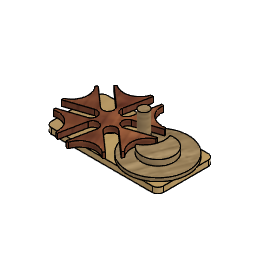
Mechanism v1 (Autodesk Fusion 360 design; units mm, degrees)
Autodesk Fusion 360 part; units mm, degrees
sketch "Sketch1" plane through (0, 0, 0) normal (0, 0, 1) x (1, 0, 0)
  line L0 (-45, 25) -> (45, 25)
  line L1 (50, 20) -> (50, -20)
  line L2 (45, -25) -> (-45, -25)
  line L3 (-50, -20) -> (-50, 20)
  arc A0 (-45, 25) -> (-50, 20) centre (-45, 20) ccw
  arc A1 (50, 20) -> (45, 25) centre (45, 20) ccw
  arc A2 (45, -25) -> (50, -20) centre (45, -20) ccw
  arc A3 (-50, -20) -> (-45, -25) centre (-45, -20) ccw
  dimension "d1" = 5
  constraint horizontal L0
  constraint vertical L1
  constraint horizontal L2
  constraint vertical L3
  constraint tangent L0 A0
  constraint tangent L3 A0
  constraint tangent L0 A1
  constraint tangent L1 A1
  constraint equal A0 A1
  constraint tangent L1 A2
  constraint tangent L2 A2
  constraint equal A0 A2
  constraint tangent L2 A3
  constraint tangent L3 A3
  constraint equal A0 A3
  measures "d1" radius of A0
extrude "Extrude1" add sketch "Sketch1" along normal blind 5 makes body 1
sketch "Sketch2" plane through (0, 0, 5) normal (0, 0, 1) x (-1, 0, 0)
  arc A0 (45, -25) -> (50, -20) centre (45, -20) ccw
  line L0 (50, -20) -> (50, 20)
  arc A1 (50, 20) -> (45, 25) centre (45, 20) ccw
  line L1 (45, 25) -> (-45, 25)
  arc A2 (-45, 25) -> (-50, 20) centre (-45, 20) ccw
  line L2 (-50, 20) -> (-50, -20)
  arc A3 (-50, -20) -> (-45, -25) centre (-45, -20) ccw
  line L3 (-45, -25) -> (45, -25)
  circle A4 centre (-25, 0) radius 27.2029
extrude "Extrude1'" add sketch "Sketch2" along normal blind 3 separate body contours L3 A4 | L1 L2 L3 A4 | L2 A4 | L1 A4 makes body 2 in component "Crank"
sketch "Sketch3" plane through (0, 0, 8) normal (0, 0, 1) x (-1, 0, 0)
  circle A0 centre (-25, 0) radius 27.2029
  circle A1 centre (-25, 0) radius 14.3178
  circle A2 centre (-47, 0) radius 15.6525
  constraint concentric A0 A1
extrude "Extrude2" add sketch "Sketch3" along normal blind 5 contours A1 A2 picked at (-24.968, 2.7723) bodies 2 in component "Crank"
sketch "Sketch4" plane through (0, 0, 8) normal (0, 0, 1) x (-1, 0, 0)
  arc A0 (-35.0909, -10.1574) -> (-35.0909, 10.1574) centre (-47, 0) ccw
  arc A1 (-35.0909, -10.1574) -> (-35.0909, 10.1574) centre (-25, 0) ccw
  circle A2 centre (-25, 0) radius 27.2029
  circle A3 centre (-47, 0) radius 4.5
  dimension "d8" = 9
  constraint concentric A0 A3
  measures "d8" diameter of A3
sketch "Sketch5" plane through (0, 0, 8) normal (0, 0, 1) x (-1, 0, 0)
extrude "Extrude3" add sketch "Sketch4" along normal blind 20 contours A3 bodies 2 in component "Crank"
sketch "Sketch1 (2)" plane through (0, 0, 5) normal (0, 0, -1) x (1, 0, 0) in component "Crank"
  circle A0 centre (25, 0) radius 27.2029
  circle A1 centre (25, 0) radius 3.6056
  constraint concentric A0 A1
extrude "Extrude4" add sketch "Sketch1 (2)" along normal blind 3 contours A1 bodies 2 in component "Crank"
sketch "Sketch2 (2)" plane through (0, 0, 5) normal (0, 0, 1) x (-1, 0, 0) in component "Crank"
  arc A0 (45, -25) -> (50, -20) centre (45, -20) ccw
  line L0 (50, -20) -> (50, 20)
  arc A1 (50, 20) -> (45, 25) centre (45, 20) ccw
  line L1 (45, 25) -> (-45, 25)
  arc A2 (-45, 25) -> (-50, 20) centre (-45, 20) ccw
  line L2 (-50, 20) -> (-50, -20)
  arc A3 (-50, -20) -> (-45, -25) centre (-45, -20) ccw
  line L3 (-45, -25) -> (45, -25)
  circle A4 centre (-25, 0) radius 5
extrude "Extrude2'" cut sketch "Sketch2 (2)" against normal blind 3 contours A4 bodies 1
extrude "Extrude5" cut sketch "Sketch2 (2)" against normal blind 3 contours A4 bodies 2 in component "Crank"
sketch "Sketch6" plane through (0, 0, 8) normal (0, 0, 1) x (-1, 0, 0)
  circle A0 centre (-47, 0) radius 4.5
  arc A1 (-35.0909, -10.1574) -> (-35.0909, 10.1574) centre (-47, 0) ccw
  arc A2 (-35.0909, -10.1574) -> (-35.0909, 10.1574) centre (-25, 0) ccw
  circle A3 centre (-25, 0) radius 27.2029
  circle A4 centre (15, 0) radius 36.685
  circle A5 centre (-6.0882, -30.018) radius 36.685
  circle A6 centre (30.4523, -33.2719) radius 36.685
  circle A7 centre (51.5405, -3.2539) radius 36.685
  circle A8 centre (36.0882, 30.018) radius 36.685
  circle A9 centre (-0.4523, 33.2719) radius 36.685
  circle A10 centre (-21.5405, 3.2539) radius 36.685
  line L0 (-6.0882, -30.018) -> (15, 0)
  line L1 (30.4523, -33.2719) -> (15, 0)
  line L2 (51.5405, -3.2539) -> (15, 0)
  line L3 (36.0882, 30.018) -> (15, 0)
  line L4 (-0.4523, 33.2719) -> (15, 0)
  line L5 (-21.5405, 3.2539) -> (15, 0)
  line L6 (-21.9839, -1.7264) -> (1.7355, -3.8386)
  arc A11 (1.7355, -3.8386) -> (2.6225, 6.122) centre (2.179, 1.1417) ccw
  line L7 (2.6225, 6.122) -> (-21.097, 8.2342)
  arc A12 (-21.097, 8.2342) -> (-21.9839, -1.7264) centre (-21.5405, 3.2539) ccw
  line L8 (-21.5405, 3.2539) -> (2.179, 1.1417) construction
  line L9 (-1.9969, -32.8922) -> (11.6379, -13.4839)
  arc A13 (11.6379, -13.4839) -> (3.4552, -7.7354) centre (7.5465, -10.6096) ccw
  line L10 (3.4552, -7.7354) -> (-10.1795, -27.1438)
  arc A14 (-10.1795, -27.1438) -> (-1.9969, -32.8922) centre (-6.0882, -30.018) ccw
  line L11 (-6.0882, -30.018) -> (7.5465, -10.6096) construction
  line L12 (34.9871, -31.1658) -> (24.9963, -9.6536)
  arc A15 (24.9963, -9.6536) -> (15.9267, -13.8658) centre (20.4615, -11.7597) ccw
  line L13 (15.9267, -13.8658) -> (25.9175, -35.378)
  arc A16 (25.9175, -35.378) -> (34.9871, -31.1658) centre (30.4523, -33.2719) ccw
  line L14 (30.4523, -33.2719) -> (20.4615, -11.7597) construction
  line L15 (51.9839, 1.7264) -> (28.3584, 3.8302)
  arc A17 (28.3584, 3.8302) -> (27.4715, -6.1304) centre (27.9149, -1.1501) ccw
  line L16 (27.4715, -6.1304) -> (51.097, -8.2342)
  arc A18 (51.097, -8.2342) -> (51.9839, 1.7264) centre (51.5405, -3.2539) ccw
  line L17 (51.5405, -3.2539) -> (27.9149, -1.1501) construction
  line L18 (31.9969, 32.8922) -> (18.3621, 13.4839)
  arc A19 (18.3621, 13.4839) -> (26.5448, 7.7354) centre (22.4535, 10.6096) ccw
  line L19 (26.5448, 7.7354) -> (40.1795, 27.1438)
  arc A20 (40.1795, 27.1438) -> (31.9969, 32.8922) centre (36.0882, 30.018) ccw
  line L20 (36.0882, 30.018) -> (22.4535, 10.6096) construction
  line L21 (-4.9871, 31.1658) -> (5.0037, 9.6536)
  arc A21 (5.0037, 9.6536) -> (14.0733, 13.8658) centre (9.5385, 11.7597) ccw
  line L22 (14.0733, 13.8658) -> (4.0825, 35.378)
  arc A22 (4.0825, 35.378) -> (-4.9871, 31.1658) centre (-0.4523, 33.2719) ccw
  line L23 (-0.4523, 33.2719) -> (9.5385, 11.7597) construction
  dimension "d17" = 10
  dimension "d18" = 23.719
  dimension "d19" = 10
  dimension "d20" = 10
  dimension "d21" = 10
  dimension "d22" = 10
  dimension "d23" = 23.719
  dimension "d24" = 10
  constraint coincident A4 A5.centre
  constraint coincident A4.centre A5
  constraint coincident A4 A6.centre
  constraint coincident A5 A6.centre
  constraint coincident A4.centre A6
  constraint coincident A4 A7.centre
  constraint coincident A6 A7.centre
  constraint coincident A4.centre A7
  constraint coincident A4 A8.centre
  constraint coincident A7 A8.centre
  constraint coincident A4.centre A8
  constraint coincident A8 A9.centre
  constraint coincident A4 A9.centre
  constraint coincident A4.centre A9
  constraint coincident A4 A10.centre
  constraint coincident A5 A10.centre
  constraint coincident A4.centre A10
  constraint coincident A5.centre L0.start
  constraint coincident A4.centre L0.end
  constraint coincident A6.centre L1.start
  constraint coincident A7.centre L2.start
  constraint coincident A8.centre L3.start
  constraint coincident A9.centre L4.start
  constraint coincident A10.centre L5.start
  constraint tangent L6 A11
  constraint tangent A11 L7
  constraint parallel L6 L7
  constraint tangent L7 A12
  constraint tangent L6 A12
  constraint coincident L5 A11.centre
  constraint coincident A3 A11.centre
  constraint parallel L5 L8
  constraint tangent L9 A13
  constraint tangent A13 L10
  constraint parallel L9 L10
  constraint tangent L10 A14
  constraint tangent L9 A14
  constraint coincident L0 A13.centre
  constraint parallel L0 L11
  constraint tangent L12 A15
  constraint tangent A15 L13
  constraint parallel L12 L13
  constraint tangent L13 A16
  constraint tangent L12 A16
  constraint parallel L1 L14
  constraint tangent L15 A17
  constraint tangent A17 L16
  constraint parallel L15 L16
  constraint tangent L16 A18
  constraint tangent L15 A18
  constraint parallel L2 L17
  constraint tangent L18 A19
  constraint tangent A19 L19
  constraint parallel L18 L19
  constraint tangent L19 A20
  constraint tangent L18 A20
  constraint parallel L3 L20
  constraint tangent L21 A21
  constraint tangent A21 L22
  constraint parallel L21 L22
  constraint tangent L22 A22
  constraint tangent L21 A22
  constraint coincident L4 A21.centre
  constraint parallel L4 L23
  measures "d17" diameter of A11
  measures "d18" distance of A5.centre A13.centre
  measures "d19" diameter of A13
  measures "d20" diameter of A15
  measures "d21" diameter of A17
  measures "d22" diameter of A19
  measures "d23" distance of A9.centre A21.centre
  measures "d24" diameter of A21
extrude "Extrude1''" add sketch "Sketch6" along normal blind 5 separate body contours A2 A4 L6 | A2 A3 A4 L6 A11 | A3 A4 A6 A9 A11 A13 L10 | A2 A3 A4 L7 | A2 A4 L7 | A3 A4 A5 A8 A11 L7 L21 A21 | A9 L5 A11 | A4 A5 A8 L12 A15 A17 L16 | A5 L5 A11 | A4 A6 A9 L15 A17 A19 L19 | A6 L0 A13 | A4 A7 A10 L18 A19 A21 L22 | A7 L1 A15 | A8 L2 A17 | A9 L3 A19 | A10 L4 A21 | A4 A7 A10 L9 A13 A15 L13 | A10 L0 A13 | A5 L1 A15 | A6 L2 A17 | A7 L3 A19 | A8 L4 A21 picked at (10.2053, -3.8088) picked at (15.9012, -6.0568) picked at (20.6959, -2.2479) picked at (19.7947, 3.8088) picked at (13.9503, 5.3986) picked at (13.0428, -5.8022) picked at (19.0463, -4.5961) picked at (21.0035, 1.2061) picked at (16.9572, 5.8022) picked at (10.9537, 4.5961) makes body 3 in component "Star gear"
move_body "Move1" bodies 3 to x (1, 0, 0) y (0, 1, 0) z (0, 0, 1) at (-3, 0, 0) in component "Star gear"
move_body "Move2" bodies 3 to x (0.906308, -0.422618, 0) y (0.422618, 0.906308, 0) z (0, 0, 1) at (-1.6865, -7.6071, 0) in component "Star gear"
sketch "Sketch7" plane through (0, 0, 13) normal (0, 0, 1) x (-1, 0, 0)
  arc A0 (13.0563, 36.3504) -> (-10.9388, 22.5463) centre (18, 0) ccw
  line L0 (-10.9388, 22.5463) -> (9.3694, 10.7794)
  arc A1 (4.356, 2.1269) -> (9.3694, 10.7794) centre (6.8627, 6.4531) ccw
  line L1 (4.356, 2.1269) -> (-15.9522, 13.8938)
  arc A2 (-15.9522, 13.8938) -> (-15.9951, -13.7886) centre (18, 0) ccw
  line L2 (-15.9951, -13.7886) -> (4.2678, -2.1316)
  arc A3 (9.2543, -10.7996) -> (4.2678, -2.1316) centre (6.7611, -6.4656) ccw
  line L3 (9.2543, -10.7996) -> (-11.0085, -22.4566)
  arc A4 (-11.0085, -22.4566) -> (12.9437, -36.3349) centre (18, 0) ccw
  line L4 (12.9437, -36.3349) -> (12.9799, -12.9583)
  arc A5 (22.9799, -12.9738) -> (12.9799, -12.9583) centre (17.9799, -12.966) ccw
  line L5 (22.9799, -12.9738) -> (22.9437, -36.3504)
  arc A6 (22.9437, -36.3504) -> (46.9388, -22.5463) centre (18, 0) ccw
  line L6 (46.9388, -22.5463) -> (26.7122, -10.8267)
  arc A7 (31.7256, -2.1741) -> (26.7122, -10.8267) centre (29.2189, -6.5004) ccw
  line L7 (31.7256, -2.1741) -> (51.9522, -13.8938)
  arc A8 (51.9522, -13.8938) -> (51.9951, 13.7886) centre (18, 0) ccw
  line L8 (51.9951, 13.7886) -> (31.7322, 2.1316)
  arc A9 (26.7457, 10.7996) -> (31.7322, 2.1316) centre (29.2389, 6.4656) ccw
  line L9 (26.7457, 10.7996) -> (47.0085, 22.4566)
  arc A10 (47.0085, 22.4566) -> (23.0563, 36.3349) centre (18, 0) ccw
  line L10 (23.0563, 36.3349) -> (23.0201, 12.9583)
  arc A11 (13.0201, 12.9738) -> (23.0201, 12.9583) centre (18.0201, 12.966) ccw
  line L11 (13.0201, 12.9738) -> (13.0563, 36.3504)
  circle A12 centre (-10.587, 0.0568) radius 14.6
  circle A13 centre (-25.1869, 0.0083) radius 14.6433
  circle A14 centre (18, 0) radius 36.685
  dimension "d27" = 29.2
  constraint coincident A12 A13.centre
  constraint concentric A0 A14
  measures "d27" diameter of A12
extrude "Extrude2''" cut sketch "Sketch7" against normal blind 5 contours A2 A13 A14 bodies 3 in component "Star gear"
move_body "Move3" bodies 3 to x (0.5, 0.866025, 0) y (-0.866025, 0.5, 0) z (0, 0, 1) at (-9, 15.5885, 0) in component "Star gear"
sketch "Sketch8" plane through (0, 0, 13) normal (0, 0, 1) x (-1, 0, 0)
  arc A0 (10.9765, -36.0064) -> (-9.68, -24.0751) centre (-3.6007, -37.3968) ccw
  arc A1 (10.9765, -36.0064) -> (12.9437, -36.3349) centre (18, 0) ccw
  line L0 (12.9437, -36.3349) -> (12.9799, -12.9583)
  arc A2 (22.9799, -12.9738) -> (12.9799, -12.9583) centre (17.9799, -12.966) ccw
  line L1 (22.9799, -12.9738) -> (22.9437, -36.3504)
  arc A3 (22.9437, -36.3504) -> (46.9388, -22.5463) centre (18, 0) ccw
  line L2 (46.9388, -22.5463) -> (26.7122, -10.8267)
  arc A4 (31.7256, -2.1741) -> (26.7122, -10.8267) centre (29.2189, -6.5004) ccw
  line L3 (31.7256, -2.1741) -> (51.9522, -13.8938)
  arc A5 (51.9522, -13.8938) -> (51.9951, 13.7886) centre (18, 0) ccw
  line L4 (51.9951, 13.7886) -> (31.7322, 2.1316)
  arc A6 (26.7457, 10.7996) -> (31.7322, 2.1316) centre (29.2389, 6.4656) ccw
  line L5 (26.7457, 10.7996) -> (47.0085, 22.4566)
  arc A7 (47.0085, 22.4566) -> (23.0563, 36.3349) centre (18, 0) ccw
  line L6 (23.0563, 36.3349) -> (23.0201, 12.9583)
  arc A8 (13.0201, 12.9738) -> (23.0201, 12.9583) centre (18.0201, 12.966) ccw
  line L7 (13.0201, 12.9738) -> (13.0563, 36.3504)
  arc A9 (13.0563, 36.3504) -> (-10.9388, 22.5463) centre (18, 0) ccw
  line L8 (-10.9388, 22.5463) -> (9.2878, 10.8267)
  arc A10 (4.2744, 2.1741) -> (9.2878, 10.8267) centre (6.7811, 6.5004) ccw
  line L9 (4.2744, 2.1741) -> (-15.9522, 13.8938)
  arc A11 (-15.9522, 13.8938) -> (-15.9951, -13.7886) centre (18, 0) ccw
  line L10 (-15.9951, -13.7886) -> (4.3495, -2.0846)
  arc A12 (9.3361, -10.7526) -> (4.3495, -2.0846) centre (6.8428, -6.4186) ccw
  line L11 (9.3361, -10.7526) -> (-11.0085, -22.4566)
  arc A13 (-11.0085, -22.4566) -> (-9.68, -24.0751) centre (18, 0) ccw
  circle A14 centre (-10.7, 0) radius 14.6
  circle A15 centre (-25.2997, -0.0928) radius 14.75
  dimension "d30" = 29.2
  dimension "d31" = 29.5
  constraint coincident A14 A15.centre
  measures "d30" diameter of A14
  measures "d31" diameter of A15
extrude "Extrude3'" cut sketch "Sketch8" against normal blind 5 contours A11 A15 bodies 3 in component "Star gear"
move_body "Move4" bodies 3 to x (0.5, 0.866025, 0) y (-0.866025, 0.5, 0) z (0, 0, 1) at (-9, 15.5885, 0) in component "Star gear"
sketch "Sketch9" plane through (0, 0, 13) normal (0, 0, 1) x (-1, 0, 0)
  arc A0 (11.1026, -36.0308) -> (-9.6518, -24.1075) centre (-3.5695, -37.545) ccw
  arc A1 (11.1026, -36.0308) -> (12.9437, -36.3349) centre (18, 0) ccw
  line L0 (12.9437, -36.3349) -> (12.9801, -12.864)
  arc A2 (22.9801, -12.8795) -> (12.9801, -12.864) centre (17.9801, -12.8717) ccw
  line L1 (22.9801, -12.8795) -> (22.9437, -36.3504)
  arc A3 (22.9437, -36.3504) -> (25.0097, -36.0091) centre (18, 0) ccw
  arc A4 (45.6707, -24.0858) -> (25.0097, -36.0091) centre (39.5862, -37.4051) ccw
  arc A5 (45.6707, -24.0858) -> (46.9388, -22.5463) centre (18, 0) ccw
  line L2 (46.9388, -22.5463) -> (26.7122, -10.8267)
  arc A6 (31.7256, -2.1741) -> (26.7122, -10.8267) centre (29.2189, -6.5004) ccw
  line L3 (31.7256, -2.1741) -> (51.9522, -13.8938)
  arc A7 (51.9522, -13.8938) -> (51.9951, 13.7886) centre (18, 0) ccw
  line L4 (51.9951, 13.7886) -> (31.7322, 2.1316)
  arc A8 (26.7457, 10.7996) -> (31.7322, 2.1316) centre (29.2389, 6.4656) ccw
  line L5 (26.7457, 10.7996) -> (47.0085, 22.4566)
  arc A9 (47.0085, 22.4566) -> (23.0563, 36.3349) centre (18, 0) ccw
  line L6 (23.0563, 36.3349) -> (23.0201, 12.9583)
  arc A10 (13.0201, 12.9738) -> (23.0201, 12.9583) centre (18.0201, 12.966) ccw
  line L7 (13.0201, 12.9738) -> (13.0563, 36.3504)
  arc A11 (13.0563, 36.3504) -> (-10.9388, 22.5463) centre (18, 0) ccw
  line L8 (-10.9388, 22.5463) -> (9.2878, 10.8267)
  arc A12 (4.2744, 2.1741) -> (9.2878, 10.8267) centre (6.7811, 6.5004) ccw
  line L9 (4.2744, 2.1741) -> (-15.9522, 13.8938)
  arc A13 (-15.9522, 13.8938) -> (-15.9951, -13.7886) centre (18, 0) ccw
  line L10 (-15.9951, -13.7886) -> (4.2678, -2.1316)
  arc A14 (9.2543, -10.7996) -> (4.2678, -2.1316) centre (6.7611, -6.4656) ccw
  line L11 (9.2543, -10.7996) -> (-11.0085, -22.4566)
  arc A15 (-11.0085, -22.4566) -> (-9.6518, -24.1075) centre (18, 0) ccw
  circle A16 centre (-24.9492, 0.0568) radius 14.5
  dimension "d34" = 29
  measures "d34" diameter of A16
extrude "Extrude4'" cut sketch "Sketch9" against normal blind 5 contours A13 A16 picked at (-15.8862, 0.0512) bodies 3 in component "Star gear"
move_body "Move5" bodies 3 to x (0.5, 0.866025, 0) y (-0.866025, 0.5, 0) z (0, 0, 1) at (-9, 15.5885, 0) in component "Star gear"
sketch "Sketch10" plane through (0, 0, 13) normal (0, 0, 1) x (-1, 0, 0)
  arc A0 (10.929, -35.9971) -> (-9.7026, -24.0491) centre (-3.5238, -37.1667) ccw
  arc A1 (10.929, -35.9971) -> (12.9437, -36.3349) centre (18, 0) ccw
  line L0 (12.9437, -36.3349) -> (12.9799, -12.9583)
  arc A2 (22.9799, -12.9738) -> (12.9799, -12.9583) centre (17.9799, -12.966) ccw
  line L1 (22.9799, -12.9738) -> (22.9437, -36.3504)
  arc A3 (22.9437, -36.3504) -> (25.0518, -36.0009) centre (18, 0) ccw
  arc A4 (45.7549, -23.9887) -> (25.0518, -36.0009) centre (39.7302, -37.4522) ccw
  arc A5 (45.7549, -23.9887) -> (46.9388, -22.5463) centre (18, 0) ccw
  line L2 (46.9388, -22.5463) -> (26.6306, -10.7794)
  arc A6 (31.644, -2.1269) -> (26.6306, -10.7794) centre (29.1373, -6.4531) ccw
  line L3 (31.644, -2.1269) -> (51.9522, -13.8938)
  arc A7 (51.9522, -13.8938) -> (52.6896, -11.934) centre (18, 0) ccw
  arc A8 (52.6942, 11.9206) -> (52.6896, -11.934) centre (61.1869, -0.0083) ccw
  arc A9 (52.6942, 11.9206) -> (51.9951, 13.7886) centre (18, 0) ccw
  line L4 (51.9951, 13.7886) -> (31.7322, 2.1316)
  arc A10 (26.7457, 10.7996) -> (31.7322, 2.1316) centre (29.2389, 6.4656) ccw
  line L5 (26.7457, 10.7996) -> (47.0085, 22.4566)
  arc A11 (47.0085, 22.4566) -> (23.0563, 36.3349) centre (18, 0) ccw
  line L6 (23.0563, 36.3349) -> (23.0201, 12.9583)
  arc A12 (13.0201, 12.9738) -> (23.0201, 12.9583) centre (18.0201, 12.966) ccw
  line L7 (13.0201, 12.9738) -> (13.0563, 36.3504)
  arc A13 (13.0563, 36.3504) -> (-10.9388, 22.5463) centre (18, 0) ccw
  line L8 (-10.9388, 22.5463) -> (9.2878, 10.8267)
  arc A14 (4.2744, 2.1741) -> (9.2878, 10.8267) centre (6.7811, 6.5004) ccw
  line L9 (4.2744, 2.1741) -> (-15.9522, 13.8938)
  arc A15 (-15.9522, 13.8938) -> (-15.9951, -13.7886) centre (18, 0) ccw
  line L10 (-15.9951, -13.7886) -> (4.2678, -2.1316)
  arc A16 (9.2543, -10.7996) -> (4.2678, -2.1316) centre (6.7611, -6.4656) ccw
  line L11 (9.2543, -10.7996) -> (-11.0085, -22.4566)
  arc A17 (-11.0085, -22.4566) -> (-9.7026, -24.0491) centre (18, 0) ccw
  circle A18 centre (-25, 0) radius 14.5
  dimension "d37" = 29
  measures "d37" diameter of A18
extrude "Extrude5'" cut sketch "Sketch10" against normal blind 5 contours A15 A18 picked at (-15.9034, 0) bodies 3 in component "Star gear"
move_body "Move6" bodies 3 to x (0.5, 0.866025, 0) y (-0.866025, 0.5, 0) z (0, 0, 1) at (-9, 15.5885, 0) in component "Star gear"
sketch "Sketch11" plane through (0, 0, 13) normal (0, 0, 1) x (-1, 0, 0)
  arc A0 (10.947, -36.0007) -> (-9.651, -24.1084) centre (-3.5, -37.2391) ccw
  arc A1 (10.947, -36.0007) -> (12.9437, -36.3349) centre (18, 0) ccw
  line L0 (12.9437, -36.3349) -> (12.9799, -12.9583)
  arc A2 (22.9799, -12.9738) -> (12.9799, -12.9583) centre (17.9799, -12.966) ccw
  line L1 (22.9799, -12.9738) -> (22.9437, -36.3504)
  arc A3 (22.9437, -36.3504) -> (24.9758, -36.0157) centre (18, 0) ccw
  arc A4 (45.6389, -24.1222) -> (24.9758, -36.0157) centre (39.4254, -37.2235) ccw
  arc A5 (45.6389, -24.1222) -> (46.9388, -22.5463) centre (18, 0) ccw
  line L2 (46.9388, -22.5463) -> (26.7122, -10.8267)
  arc A6 (31.7256, -2.1741) -> (26.7122, -10.8267) centre (29.2189, -6.5004) ccw
  line L3 (31.7256, -2.1741) -> (51.9522, -13.8938)
  arc A7 (51.9522, -13.8938) -> (52.7036, -11.8934) centre (18, 0) ccw
  arc A8 (52.6523, 12.0421) -> (52.7036, -11.8934) centre (61.2997, 0.0928) ccw
  arc A9 (52.6523, 12.0421) -> (51.9951, 13.7886) centre (18, 0) ccw
  line L4 (51.9951, 13.7886) -> (31.6505, 2.0846)
  arc A10 (26.6639, 10.7526) -> (31.6505, 2.0846) centre (29.1572, 6.4186) ccw
  line L5 (26.6639, 10.7526) -> (47.0085, 22.4566)
  arc A11 (47.0085, 22.4566) -> (45.68, 24.0751) centre (18, 0) ccw
  arc A12 (25.0235, 36.0064) -> (45.68, 24.0751) centre (39.6007, 37.3968) ccw
  arc A13 (25.0235, 36.0064) -> (23.0563, 36.3349) centre (18, 0) ccw
  line L6 (23.0563, 36.3349) -> (23.0201, 12.9583)
  arc A14 (13.0201, 12.9738) -> (23.0201, 12.9583) centre (18.0201, 12.966) ccw
  line L7 (13.0201, 12.9738) -> (13.0563, 36.3504)
  arc A15 (13.0563, 36.3504) -> (-10.9388, 22.5463) centre (18, 0) ccw
  line L8 (-10.9388, 22.5463) -> (9.2878, 10.8267)
  arc A16 (4.2744, 2.1741) -> (9.2878, 10.8267) centre (6.7811, 6.5004) ccw
  line L9 (4.2744, 2.1741) -> (-15.9522, 13.8938)
  arc A17 (-15.9522, 13.8938) -> (-15.9951, -13.7886) centre (18, 0) ccw
  line L10 (-15.9951, -13.7886) -> (4.2678, -2.1316)
  arc A18 (9.2543, -10.7996) -> (4.2678, -2.1316) centre (6.7611, -6.4656) ccw
  line L11 (9.2543, -10.7996) -> (-11.0085, -22.4566)
  arc A19 (-11.0085, -22.4566) -> (-9.651, -24.1084) centre (18, 0) ccw
  circle A20 centre (-25, 0) radius 14.5
  dimension "d40" = 29
  measures "d40" diameter of A20
extrude "Extrude6" cut sketch "Sketch11" against normal blind 5 contours A17 A20 picked at (-15.9034, 0) bodies 3 in component "Star gear"
move_body "Move7" bodies 3 to x (0.5, 0.866025, 0) y (-0.866025, 0.5, 0) z (0, 0, 1) at (-9, 15.5885, 0) in component "Star gear"
sketch "Sketch12" plane through (0, 0, 13) normal (0, 0, 1) x (-1, 0, 0)
  arc A0 (10.947, -36.0007) -> (-9.651, -24.1084) centre (-3.5, -37.2391) ccw
  arc A1 (10.947, -36.0007) -> (12.9437, -36.3349) centre (18, 0) ccw
  line L0 (12.9437, -36.3349) -> (12.9799, -12.9583)
  arc A2 (22.9799, -12.9738) -> (12.9799, -12.9583) centre (17.9799, -12.966) ccw
  line L1 (22.9799, -12.9738) -> (22.9437, -36.3504)
  arc A3 (22.9437, -36.3504) -> (25.053, -36.0007) centre (18, 0) ccw
  arc A4 (45.651, -24.1084) -> (25.053, -36.0007) centre (39.5, -37.2391) ccw
  arc A5 (45.651, -24.1084) -> (46.9388, -22.5463) centre (18, 0) ccw
  line L2 (46.9388, -22.5463) -> (26.7122, -10.8267)
  arc A6 (31.7256, -2.1741) -> (26.7122, -10.8267) centre (29.2189, -6.5004) ccw
  line L3 (31.7256, -2.1741) -> (51.9522, -13.8938)
  arc A7 (51.9522, -13.8938) -> (52.6784, -11.9666) centre (18, 0) ccw
  arc A8 (52.7099, 11.8749) -> (52.6784, -11.9666) centre (60.9492, -0.0568) ccw
  arc A9 (52.7099, 11.8749) -> (51.9951, 13.7886) centre (18, 0) ccw
  line L4 (51.9951, 13.7886) -> (31.7322, 2.1316)
  arc A10 (26.7457, 10.7996) -> (31.7322, 2.1316) centre (29.2389, 6.4656) ccw
  line L5 (26.7457, 10.7996) -> (47.0085, 22.4566)
  arc A11 (47.0085, 22.4566) -> (45.6518, 24.1075) centre (18, 0) ccw
  arc A12 (24.8974, 36.0308) -> (45.6518, 24.1075) centre (39.5695, 37.545) ccw
  arc A13 (24.8974, 36.0308) -> (23.0563, 36.3349) centre (18, 0) ccw
  line L6 (23.0563, 36.3349) -> (23.0199, 12.864)
  arc A14 (13.0199, 12.8795) -> (23.0199, 12.864) centre (18.0199, 12.8717) ccw
  line L7 (13.0199, 12.8795) -> (13.0563, 36.3504)
  arc A15 (13.0563, 36.3504) -> (10.9903, 36.0091) centre (18, 0) ccw
  arc A16 (-9.6707, 24.0858) -> (10.9903, 36.0091) centre (-3.5862, 37.4051) ccw
  arc A17 (-9.6707, 24.0858) -> (-10.9388, 22.5463) centre (18, 0) ccw
  line L8 (-10.9388, 22.5463) -> (9.2878, 10.8267)
  arc A18 (4.2744, 2.1741) -> (9.2878, 10.8267) centre (6.7811, 6.5004) ccw
  line L9 (4.2744, 2.1741) -> (-15.9522, 13.8938)
  arc A19 (-15.9522, 13.8938) -> (-15.9951, -13.7886) centre (18, 0) ccw
  line L10 (-15.9951, -13.7886) -> (4.2678, -2.1316)
  arc A20 (9.2543, -10.7996) -> (4.2678, -2.1316) centre (6.7611, -6.4656) ccw
  line L11 (9.2543, -10.7996) -> (-11.0085, -22.4566)
  arc A21 (-11.0085, -22.4566) -> (-9.651, -24.1084) centre (18, 0) ccw
  circle A22 centre (-25, 0) radius 14.5
  dimension "d43" = 29
  measures "d43" diameter of A22
extrude "Extrude7" cut sketch "Sketch12" against normal blind 5 contours A19 A22 picked at (-15.9034, 0) bodies 3 in component "Star gear"
sketch "Sketch13" plane through (0, 0, 8) normal (0, 0, -1) x (1, 0, 0)
  arc A0 (16.704, 11.8923) -> (16.704, -11.8923) centre (25, 0) ccw
  arc A1 (16.704, 11.8923) -> (15.9522, 13.8938) centre (-18, 0) ccw
  line L0 (15.9522, 13.8938) -> (-4.2744, 2.1741)
  arc A2 (-9.2878, 10.8267) -> (-4.2744, 2.1741) centre (-6.7811, 6.5004) ccw
  line L1 (-9.2878, 10.8267) -> (10.9388, 22.5463)
  arc A3 (10.9388, 22.5463) -> (9.6707, 24.0858) centre (-18, 0) ccw
  arc A4 (-10.9903, 36.0091) -> (9.6707, 24.0858) centre (3.5862, 37.4051) ccw
  arc A5 (-10.9903, 36.0091) -> (-13.0563, 36.3504) centre (-18, 0) ccw
  line L2 (-13.0563, 36.3504) -> (-13.0199, 12.8795)
  arc A6 (-23.0199, 12.864) -> (-13.0199, 12.8795) centre (-18.0199, 12.8717) ccw
  line L3 (-23.0199, 12.864) -> (-23.0563, 36.3349)
  arc A7 (-23.0563, 36.3349) -> (-24.8974, 36.0308) centre (-18, 0) ccw
  arc A8 (-45.6518, 24.1075) -> (-24.8974, 36.0308) centre (-39.5695, 37.545) ccw
  arc A9 (-45.6518, 24.1075) -> (-47.0085, 22.4566) centre (-18, 0) ccw
  line L4 (-47.0085, 22.4566) -> (-26.7457, 10.7996)
  arc A10 (-31.7322, 2.1316) -> (-26.7457, 10.7996) centre (-29.2389, 6.4656) ccw
  line L5 (-31.7322, 2.1316) -> (-51.9951, 13.7886)
  arc A11 (-51.9951, 13.7886) -> (-52.7099, 11.8749) centre (-18, 0) ccw
  arc A12 (-52.6784, -11.9666) -> (-52.7099, 11.8749) centre (-60.9492, -0.0568) ccw
  arc A13 (-52.6784, -11.9666) -> (-51.9522, -13.8938) centre (-18, 0) ccw
  line L6 (-51.9522, -13.8938) -> (-31.7256, -2.1741)
  arc A14 (-26.7122, -10.8267) -> (-31.7256, -2.1741) centre (-29.2189, -6.5004) ccw
  line L7 (-26.7122, -10.8267) -> (-46.9388, -22.5463)
  arc A15 (-46.9388, -22.5463) -> (-45.651, -24.1084) centre (-18, 0) ccw
  arc A16 (-25.053, -36.0007) -> (-45.651, -24.1084) centre (-39.5, -37.2391) ccw
  arc A17 (-25.053, -36.0007) -> (-22.9437, -36.3504) centre (-18, 0) ccw
  line L8 (-22.9437, -36.3504) -> (-22.9799, -12.9738)
  arc A18 (-12.9799, -12.9583) -> (-22.9799, -12.9738) centre (-17.9799, -12.966) ccw
  line L9 (-12.9799, -12.9583) -> (-12.9437, -36.3349)
  arc A19 (-12.9437, -36.3349) -> (-10.947, -36.0007) centre (-18, 0) ccw
  arc A20 (9.651, -24.1084) -> (-10.947, -36.0007) centre (3.5, -37.2391) ccw
  arc A21 (9.651, -24.1084) -> (11.0085, -22.4566) centre (-18, 0) ccw
  line L10 (11.0085, -22.4566) -> (-9.2543, -10.7996)
  arc A22 (-4.2678, -2.1316) -> (-9.2543, -10.7996) centre (-6.7611, -6.4656) ccw
  line L11 (-4.2678, -2.1316) -> (15.9951, -13.7886)
  arc A23 (15.9951, -13.7886) -> (16.704, -11.8923) centre (-18, 0) ccw
  circle A24 centre (-18, 0) radius 5
  dimension "d46" = 10
  constraint concentric A1 A24
  measures "d46" diameter of A24
extrude "Extrude3''" cut sketch "Sketch13" along normal blind 6 contours A24 bodies 1
sketch "Sketch14" plane through (0, 0, 8) normal (0, 0, -1) x (1, 0, 0)
  arc A0 (16.704, 11.8923) -> (16.704, -11.8923) centre (25, 0) ccw
  arc A1 (16.704, 11.8923) -> (15.9522, 13.8938) centre (-18, 0) ccw
  line L0 (15.9522, 13.8938) -> (-4.2744, 2.1741)
  arc A2 (-9.2878, 10.8267) -> (-4.2744, 2.1741) centre (-6.7811, 6.5004) ccw
  line L1 (-9.2878, 10.8267) -> (10.9388, 22.5463)
  arc A3 (10.9388, 22.5463) -> (9.6707, 24.0858) centre (-18, 0) ccw
  arc A4 (-10.9903, 36.0091) -> (9.6707, 24.0858) centre (3.5862, 37.4051) ccw
  arc A5 (-10.9903, 36.0091) -> (-13.0563, 36.3504) centre (-18, 0) ccw
  line L2 (-13.0563, 36.3504) -> (-13.0199, 12.8795)
  arc A6 (-23.0199, 12.864) -> (-13.0199, 12.8795) centre (-18.0199, 12.8717) ccw
  line L3 (-23.0199, 12.864) -> (-23.0563, 36.3349)
  arc A7 (-23.0563, 36.3349) -> (-24.8974, 36.0308) centre (-18, 0) ccw
  arc A8 (-45.6518, 24.1075) -> (-24.8974, 36.0308) centre (-39.5695, 37.545) ccw
  arc A9 (-45.6518, 24.1075) -> (-47.0085, 22.4566) centre (-18, 0) ccw
  line L4 (-47.0085, 22.4566) -> (-26.7457, 10.7996)
  arc A10 (-31.7322, 2.1316) -> (-26.7457, 10.7996) centre (-29.2389, 6.4656) ccw
  line L5 (-31.7322, 2.1316) -> (-51.9951, 13.7886)
  arc A11 (-51.9951, 13.7886) -> (-52.7099, 11.8749) centre (-18, 0) ccw
  arc A12 (-52.6784, -11.9666) -> (-52.7099, 11.8749) centre (-60.9492, -0.0568) ccw
  arc A13 (-52.6784, -11.9666) -> (-51.9522, -13.8938) centre (-18, 0) ccw
  line L6 (-51.9522, -13.8938) -> (-31.7256, -2.1741)
  arc A14 (-26.7122, -10.8267) -> (-31.7256, -2.1741) centre (-29.2189, -6.5004) ccw
  line L7 (-26.7122, -10.8267) -> (-46.9388, -22.5463)
  arc A15 (-46.9388, -22.5463) -> (-45.651, -24.1084) centre (-18, 0) ccw
  arc A16 (-25.053, -36.0007) -> (-45.651, -24.1084) centre (-39.5, -37.2391) ccw
  arc A17 (-25.053, -36.0007) -> (-22.9437, -36.3504) centre (-18, 0) ccw
  line L8 (-22.9437, -36.3504) -> (-22.9799, -12.9738)
  arc A18 (-12.9799, -12.9583) -> (-22.9799, -12.9738) centre (-17.9799, -12.966) ccw
  line L9 (-12.9799, -12.9583) -> (-12.9437, -36.3349)
  arc A19 (-12.9437, -36.3349) -> (-10.947, -36.0007) centre (-18, 0) ccw
  arc A20 (9.651, -24.1084) -> (-10.947, -36.0007) centre (3.5, -37.2391) ccw
  arc A21 (9.651, -24.1084) -> (11.0085, -22.4566) centre (-18, 0) ccw
  line L10 (11.0085, -22.4566) -> (-9.2543, -10.7996)
  arc A22 (-4.2678, -2.1316) -> (-9.2543, -10.7996) centre (-6.7611, -6.4656) ccw
  line L11 (-4.2678, -2.1316) -> (15.9951, -13.7886)
  arc A23 (15.9951, -13.7886) -> (16.704, -11.8923) centre (-18, 0) ccw
  circle A24 centre (-18, 0) radius 4.95
  dimension "d49" = 9.9
  constraint concentric A1 A24
  measures "d49" diameter of A24
extrude "Extrude8" add sketch "Sketch14" along normal blind 6.9 contours A24 bodies 3 in component "Star gear"
sketch "Sketch15" plane through (0, 0, 5) normal (0, 0, -1) x (1, 0, 0)
  circle A0 centre (25, 0) radius 27.2029
  circle A1 centre (25, 0) radius 4.95
  dimension "d52" = 9.9
  constraint concentric A0 A1
  measures "d52" diameter of A1
extrude "Extrude6'" add sketch "Sketch15" along normal blind 2.9 contours A1 bodies 2 in component "Crank"
copy_body "Body->Comp1" bodies 1 removing the originals makes body 4 in component "Stand"
sketch "Sketch16" plane through (0, 0, 8) normal (0, 0, 1) x (-1, 0, 0)
  circle A0 centre (-47, 0) radius 4.5
  arc A1 (-35.0909, -10.1574) -> (-35.0909, 10.1574) centre (-47, 0) ccw
  arc A2 (-35.0909, -10.1574) -> (-35.0909, 10.1574) centre (-25, 0) ccw
  circle A3 centre (-25, 0) radius 27.2029
  circle A4 centre (-47, 0) radius 18.4391
  circle A5 centre (-28.5609, 0) radius 13.9391
  constraint concentric A0 A4
  constraint coincident A4 A5.centre
  constraint tangent A0 A5
extrude "Extrude7'" cut sketch "Sketch16" along normal blind 5 contours A1 A2 A4 bodies 2 in component "Crank"
component "Crank" placed x (1, 0, 0) y (0, 1, 0) z (0, 0, 1) at (0, 0, 0)
component "Star gear" placed x (1, 0, 0) y (0, 1, 0) z (0, 0, 1) at (0, 0, 0)
component "Stand" placed x (1, 0, 0) y (0, 1, 0) z (0, 0, 1) at (0, 0, 0)
